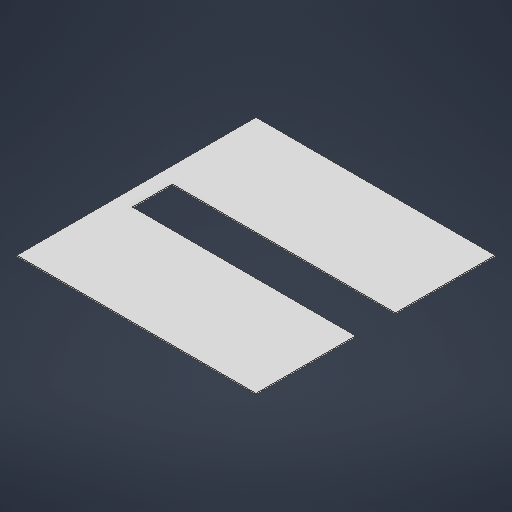
# Autodesk Inventor part: parte frontal
Saved by Autodesk Inventor 2027 (Build 310192060, 192F)
## iProperties
Created: 2026-09-04
Part Number: parte frontal
Material: Genérico
Document SubType Name: Modeling
Designer: Leandro
Density: 1 g/cm^3
Appearance: Valor por defecto
Author: Leandro
Autodesk Inventor part; units mm, degrees
ref_plane "YZ Plane" through (0, 0, 0) normal (1, 0, 0) x (0, 1, 0)
ref_plane "XZ Plane" through (0, 0, 0) normal (0, 1, 0) x (-1, 0, 0)
ref_plane "XY Plane" through (0, 0, 0) normal (0, 0, 1) x (1, 0, 0)
sketch "Boceto1" plane through (0, 0, 0) normal (0, 1, 0) x (-1, 0, 0)
  line L0 (11.9544, 13.1521) -> (-288.0456, 13.1521)
  line L1 (-288.0456, -286.8479) -> (11.9544, -286.8479)
  line L2 (11.9544, -286.8479) -> (11.9544, 13.1521)
  line L3 (-8.0456, -136.8479) -> (-8.0456, -161.8479)
  line L4 (-8.0456, -161.8479) -> (-288.0456, -161.8479)
  line L5 (-8.0456, -136.8479) -> (-8.0456, -111.8479)
  line L6 (-8.0456, -111.8479) -> (-288.0456, -111.8479)
  line L7 (-288.0456, 13.1521) -> (-288.0456, -111.8479)
  line L8 (-288.0456, -161.8479) -> (-288.0456, -286.8479)
  point P0 (0, 0)
  dimension "d0" = 300
  dimension "d1" = 300
  dimension "d3" = 25
  dimension "d4" = 25
  constraints: 18 end point, 6 perpendicular, 3 parallel, 1 horizontal
  measures "d0" distance of L1.end L1.start
  measures "d1" distance of L1.start L0.end
  measures "d3" distance of L3.start L3.end
  measures "d4" distance of L3.start L5.end
extrude "Extrusión1" add sketch "Boceto1" along normal mid plane 1.5
